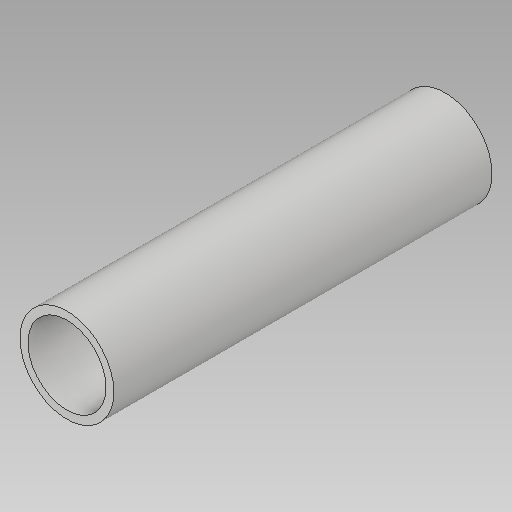
# Autodesk Inventor part: tube-13
Saved by Autodesk Inventor 2021 (Build 250183000, 183)
## iProperties
Created: 2020-04-27
Part Number: tube-13
Material: Aluminum 6061 T6 0 Cold Formed
Document SubType Name: Modeling
Designer: Hannah
Density: 2.7 g/cm^3
Appearance: Satin
length: 170.000 mm
size: 7.000 ul
Author: Hannah
Autodesk Inventor part; units mm, degrees
ref_plane "YZ Plane" through (0, 0, 0) normal (1, 0, 0) x (0, 1, 0)
ref_plane "XZ Plane" through (0, 0, 0) normal (0, 1, 0) x (-1, 0, 0)
ref_plane "XY Plane" through (0, 0, 0) normal (0, 0, 1) x (1, 0, 0)
sketch "Sketch1" plane through (0, 0, 0) normal (0, 0, 1) x (1, 0, 0)
  circle A0 centre (0, 0) radius 21.1
  circle A1 centre (0, 0) radius 17.54
  dimension "OD" = 42.2
  dimension "t" = 3.56
  constraints: 2 centre point, 2 coincident
  measures "OD" diameter of A0
  measures "t" radial gap between concentric circles of A0 A1
extrude "Extrusion1" add sketch "Sketch1" along normal mid plane 170
equation "\"size\" = 7"
body "Solid1"
